nema 17 planetray gearbox v5 (Autodesk Fusion 360 design; units mm, degrees)
Autodesk Fusion 360 part; units mm, degrees
sketch "Sketch1" plane through (0, 0, 0) normal (0, 0, 1) x (1, 0, 0)
  line L0 (16.8, 21) -> (-16.8, 21)
  line L1 (-21, 16.8) -> (-21, -16.8)
  line L2 (-16.8, -21) -> (16.8, -21)
  line L3 (21, -16.8) -> (21, 16.8)
  line L4 (21, 21) -> (-21, -21) construction
  line L5 (-21, 21) -> (21, -21) construction
  circle A0 centre (0, 0) radius 18
  line L6 (15.5, 15.5) -> (-15.5, 15.5) construction
  line L7 (-15.5, 15.5) -> (-15.5, -15.5) construction
  line L8 (-15.5, -15.5) -> (15.5, -15.5) construction
  line L9 (15.5, -15.5) -> (15.5, 15.5) construction
  line L10 (15.5, 15.5) -> (-15.5, -15.5) construction
  line L11 (-15.5, 15.5) -> (15.5, -15.5) construction
  circle A1 centre (15.5, 15.5) radius 2
  circle A2 centre (-15.5, 15.5) radius 2
  circle A3 centre (-15.5, -15.5) radius 2
  circle A4 centre (15.5, -15.5) radius 2
  line L12 (-21, 16.8) -> (-16.8, 21)
  line L13 (21, 16.8) -> (16.8, 21)
  line L14 (21, -16.8) -> (16.8, -21)
  line L15 (-16.8, -21) -> (-21, -16.8)
  dimension "d1" = 42
  dimension "d2" = 42
  dimension "d3" = 36
  dimension "d4" = 31
  dimension "d5" = 31
  dimension "d6" = 4
  dimension "d7" = 4
  dimension "d8" = 4
  dimension "d9" = 4
  dimension "d10" = 4.2
  dimension "d11" = 4.2
  dimension "d12" = 4.2
  dimension "d13" = 4.2
  dimension "d14" = 4.2
  dimension "d15" = 4.2
  dimension "d16" = 4.2
  dimension "d17" = 4.2
  constraint horizontal L0
  constraint perpendicular L0 L1
  constraint parallel L0 L2
  constraint parallel L1 L3
  constraint coincident L4 A0.centre
  constraint coincident L5 A0.centre
  constraint coincident A0.centre origin
  constraint horizontal L6
  constraint perpendicular L6 L7
  constraint parallel L6 L8
  constraint parallel L7 L9
  constraint coincident L10 A0.centre
  constraint coincident L11 A0.centre
  constraint coincident L6.start L9.end
  constraint coincident L6.end L7.start
  constraint coincident L7.end L8.start
  constraint coincident L8.end L9.start
  constraint coincident L5.start L1
  constraint coincident L5.start L0
  constraint coincident L4.start L3
  constraint coincident L4.start L0
  constraint coincident L5.end L3
  constraint coincident L5.end L2
  constraint coincident L4.end L2
  constraint coincident L4.end L1
  measures "d1" distance of L4.end L5.end
  measures "d2" distance of L5.start L4.end
  measures "d3" diameter of A0
  measures "d4" distance of L7.end L8.end
  measures "d5" distance of L6.end L7.end
  measures "d6" diameter of A1
  measures "d7" diameter of A2
  measures "d8" diameter of A3
  measures "d9" diameter of A4
  measures "d10" distance of L5.start L1.start
  measures "d11" distance of L5.start L0.end
  measures "d12" distance of L4.start L3.end
  measures "d13" distance of L4.start L0.start
  measures "d14" distance of L5.end L3.start
  measures "d15" distance of L5.end L2.end
  measures "d16" distance of L4.end L2.start
  measures "d17" distance of L4.end L1.end
extrude "Extrude1" add sketch "Sketch1" along normal blind 38.5 contours A0 makes body 1
sketch "Sketch2" plane through (0, 0, 38.5) normal (0, 0, 1) x (-1, 0, 0)
  circle A0 centre (0, 0) radius 18
  circle A1 centre (0, 0) radius 11
  dimension "d20" = 22
  constraint concentric A0 A1
  measures "d20" diameter of A1
extrude "Extrude2" add sketch "Sketch2" along normal blind 2 contours A1 bodies 1
sketch "Sketch3" plane through (0, 0, 40.5) normal (0, 0, 1) x (-1, 0, 0)
  circle A0 centre (0, 0) radius 11
  circle A1 centre (0, 0) radius 4
  line L0 (-2.6458, 3) -> (2.6458, 3)
  line L1 (-2.6458, -3) -> (2.6458, -3)
  line L2 (0, 0) -> (-4, 0) construction
  dimension "d23" = 8
  dimension "d26" = 6
  constraint coincident A0.centre A1.centre
  constraint coincident A1 L0.start
  constraint coincident A1 L0.end
  constraint horizontal L0
  constraint coincident A1 L1.start
  constraint parallel L0 L1
  constraint coincident A1 L1.end
  constraint coincident A1 L2.end
  constraint horizontal L2
  constraint symmetric L0 L1 L2
  measures "d23" diameter of A1
  measures "d26" distance of L0 L1
extrude "Extrude3" add sketch "Sketch3" along normal blind 16.5 separate body contours A1 L0 L1 makes body 2
extrude "Extrude4" add sketch "Sketch3" along normal blind 1.5 contours A1 L0 | A1 L1 bodies 2
extrude "Extrude5" add sketch "Sketch1" along normal blind 3 bodies 1
sketch "Sketch4" plane through (0, 0, 38.5) normal (0, 0, 1) x (-1, 0, 0)
  circle A0 centre (0, 0) radius 11
  circle A1 centre (0, 0) radius 18
  circle A2 centre (0, 0) radius 14 construction
  line L0 (0, 0) -> (0, 14) construction
  line L1 (0, 0) -> (-9.8995, 9.8995) construction
  line L2 (0, 14) -> (-2.8, 14) construction
  line L3 (-2.8, 14) -> (-2.8, 17.7809)
  line L4 (0, 14) -> (2.8, 14) construction
  line L5 (2.8, 14) -> (2.8, 17.7809)
  arc A3 (-2.8, 14) -> (2.8, 14) centre (0, 14) ccw
  line L6 (-14, 2.8) -> (-17.7809, 2.8)
  arc A4 (-14, -2.8) -> (-14, 2.8) centre (-14, 0) ccw
  line L7 (-14, -2.8) -> (-17.7809, -2.8)
  line L8 (-2.8, -14) -> (-2.8, -17.7809)
  arc A5 (2.8, -14) -> (-2.8, -14) centre (0, -14) ccw
  line L9 (2.8, -14) -> (2.8, -17.7809)
  line L10 (14, -2.8) -> (17.7809, -2.8)
  arc A6 (14, 2.8) -> (14, -2.8) centre (14, 0) ccw
  line L11 (14, 2.8) -> (17.7809, 2.8)
  circle A7 centre (-9.8995, 9.8995) radius 1.5
  circle A8 centre (-9.8995, -9.8995) radius 1.5
  circle A9 centre (9.8995, -9.8995) radius 1.5
  circle A10 centre (9.8995, 9.8995) radius 1.5
  dimension "d31" = 28
  dimension "d32" = 45
  dimension "d33" = 2.8
  dimension "d35" = 360
  dimension "d36" = 3
  dimension "d38" = 360
  constraint concentric A0 A2
  constraint coincident A0.centre A1.centre
  constraint coincident A2 L0.end
  constraint vertical L0
  constraint coincident A2 L1.end
  constraint coincident L0.end L2.start
  constraint tangent A2 L2
  constraint perpendicular L0 L2
  constraint coincident A1 L3.end
  constraint tangent L3 A3
  constraint tangent A2 L4
  constraint perpendicular L0 L4
  constraint coincident A1 L5.end
  constraint tangent L5 A3
  constraint coincident L1.end A7.centre
  measures "d31" diameter of A2
  measures "d32" angle of L0 L1
  measures "d33" radius of A3
  measures "d36" diameter of A7
extrude "Extrude6" cut sketch "Sketch4" against normal blind 3 contours A1 L10 A6 L11 | A1 L3 L5 A3 | A1 L8 A5 L9 | A1 L6 A4 L7 bodies 2 1
extrude "Extrude7" cut sketch "Sketch4" against normal blind 5 contours A7 | A8 | A9 | A10 bodies 2 1
sketch "Sketch5" plane through (0, 0, 35.5) normal (0, 0, 1) x (-1, 0, 0)
  arc A0 (-2.8, 14) -> (2.8, 14) centre (0, 14) ccw
  line L0 (2.8, 14) -> (2.8, 17.7809)
  arc A1 (2.8, 17.7809) -> (-2.8, 17.7809) centre (0, 0) ccw
  line L1 (-2.8, 17.7809) -> (-2.8, 14)
  line L2 (14, -2.8) -> (17.7809, -2.8)
  arc A2 (17.7809, -2.8) -> (17.7809, 2.8) centre (0, 0) ccw
  line L3 (17.7809, 2.8) -> (14, 2.8)
  arc A3 (14, 2.8) -> (14, -2.8) centre (14, 0) ccw
  line L4 (-2.8, -14) -> (-2.8, -17.7809)
  arc A4 (-2.8, -17.7809) -> (2.8, -17.7809) centre (0, 0) ccw
  line L5 (2.8, -17.7809) -> (2.8, -14)
  arc A5 (2.8, -14) -> (-2.8, -14) centre (0, -14) ccw
  line L6 (-14, 2.8) -> (-17.7809, 2.8)
  arc A6 (-17.7809, 2.8) -> (-17.7809, -2.8) centre (0, 0) ccw
  line L7 (-17.7809, -2.8) -> (-14, -2.8)
  arc A7 (-14, -2.8) -> (-14, 2.8) centre (-14, 0) ccw
  circle A8 centre (0, 0) radius 11
  circle A9 centre (0, 0) radius 14 construction
  circle A10 centre (-14, 0) radius 2.25
  circle A11 centre (0, -14) radius 2.25
  circle A12 centre (14, 0) radius 2.25
  circle A13 centre (0, 14) radius 2.25
  dimension "d43" = 4.5
  dimension "d45" = 360
  constraint concentric A4 A9
  constraint coincident A7.centre A9
  constraint concentric A7 A10
  measures "d43" diameter of A10
extrude "Extrude8" add sketch "Sketch5" along normal blind 2.5 contours A10 | A11 | A12 | A13 bodies 1 2
sketch "Sketch6" plane through (0, 0, 0) normal (0, 0, -1) x (1, 0, 0)
  line L0 (21, -16.8) -> (21, 16.8)
  line L1 (21, 16.8) -> (16.8, 21)
  line L2 (16.8, 21) -> (-16.8, 21)
  line L3 (-16.8, 21) -> (-21, 16.8)
  line L4 (-21, 16.8) -> (-21, -16.8)
  line L5 (-21, -16.8) -> (-16.8, -21)
  line L6 (-16.8, -21) -> (16.8, -21)
  line L7 (16.8, -21) -> (21, -16.8)
  circle A0 centre (-15.5, -15.5) radius 2
  circle A1 centre (15.5, -15.5) radius 2
  circle A2 centre (15.5, 15.5) radius 2
  circle A3 centre (-15.5, 15.5) radius 2
  circle A4 centre (0, 0) radius 6
  dimension "d48" = 12
  constraint coincident A4.centre origin
  measures "d48" diameter of A4
extrude "Extrude9" cut sketch "Sketch6" against normal blind 10.5 contours A4 bodies 2 1
equation "d11 = d10"
equation "d12 = d10"
equation "d13 = d12"
equation "d14 = d10"
equation "d15 = d14"
equation "d16 = d10"
equation "d17 = d16"
